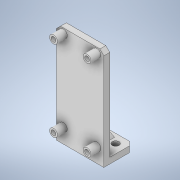
# Autodesk Inventor part: Vertical Ultrasonic Sensor Mount
Saved by Autodesk Inventor 2022.6 (Build 266554000, 554)
## iProperties
Created: 2024-10-19
Part Number: Vertical Ultrasonic Sensor Mount
Material: Generic
Document SubType Name: Modeling
Designer: Asus
Density: 1 g/cm^3
Appearance: Default
Author: Asus
Autodesk Inventor part; units mm, degrees
ref_plane "XY Plane" through (0, 0, 0) normal (0, 0, 1) x (1, 0, 0)
sketch "Sketch1" plane through (0, 0, 0) normal (0, 0, 1) x (1, 0, 0)
  line L0 (0, 0) -> (24, 0)
  line L1 (24, 0) -> (24, 46)
  line L2 (24, 46) -> (0, 46)
  line L3 (0, 46) -> (0, 0)
  line L4 (0, 46) -> (24, 46)
  line L5 (24, 46) -> (24, 46)
  line L6 (24, 46) -> (0, 46)
  line L7 (0, 46) -> (0, 46)
  dimension "d0" = 24
  dimension "d1" = 46
  dimension "d47" = 0
  dimension "d48" = 24
  constraints: 16 end point, 4 equal length, 2 horizontal, 2 perpendicular
  measures "d0" distance of L2.end L1.end
  measures "d1" distance of L1.end L0.end
  measures "d47" distance between parallel lines of L2 L6
  measures "d48" distance of L5.end L6.end
extrude "Extrusion1" add sketch "Sketch1" along normal blind 3
ref_plane "Work Plane1" through (12, 0, 0) normal (1, 0, 0) x (0, 1, 0)
ref_plane "Work Plane2" through (0, 23, 0) normal (0, 1, 0) x (-1, 0, 0)
sketch "Sketch2" plane through (0, 0, 3) normal (0, 0, 1) x (1, 0, 0)
  line L0 (24, 46) -> (0, 46) projected
  line L1 (0, 46) -> (0, 0) projected
  line L2 (24, 0) -> (24, 46) projected
  line L3 (0, 0) -> (24, 0) projected
  circle A0 centre (3.5, 43.5) radius 2
  circle A1 centre (3.5, 43.5) radius 1.2
  circle A2 centre (20.5, 43.5) radius 2
  circle A3 centre (20.5, 43.5) radius 1.2
  circle A4 centre (3.5, 2.5) radius 2
  circle A5 centre (3.5, 2.5) radius 1.2
  circle A6 centre (20.5, 2.5) radius 1.2
  circle A7 centre (20.5, 2.5) radius 2
  dimension "d4" = 17
  dimension "d6" = 41
  dimension "d7" = 2.5
  dimension "d8" = 3.5
  dimension "d11" = 3.5
  dimension "d12" = 3.5
  dimension "d13" = 2.5
  dimension "d14" = 41
  dimension "d15" = 4
  dimension "d16" = 2.4
  dimension "d17" = 4
  dimension "d18" = 2.4
  dimension "d19" = 4
  dimension "d20" = 2.4
  dimension "d21" = 2.4
  dimension "d22" = 4
  constraints: 8 centre point, 8 coincident
  measures "d4" distance of point (20.5, 43.5) point (3.5, 43.5)
  measures "d6" distance of point (3.5, 2.5) point (3.5, 43.5)
  measures "d7" distance from line of point (3.5, 43.5) L0
  measures "d8" distance from line of point (3.5, 43.5) L1
  measures "d11" distance from line of L1 point (3.5, 2.5)
  measures "d12" distance from line of L2 point (20.5, 2.5)
  measures "d13" distance from line of L3 point (20.5, 2.5)
  measures "d14" distance of point (20.5, 2.5) point (20.5, 43.5)
  measures "d15" diameter of A0
  measures "d16" diameter of A1
  measures "d17" diameter of A2
  measures "d18" diameter of A3
  measures "d19" diameter of A4
  measures "d20" diameter of A5
  measures "d21" diameter of A6
  measures "d22" diameter of A7
extrude "Extrusion2" add sketch "Sketch2" along normal blind 5 contours A0 | A2 | A4 | A7
hole "Hole1" at (3.5, 43.5, 3) at (20.5, 43.5, 3) at (3.5, 2.5, 3) at (20.5, 2.5, 3) direction (0, 0, -1) diameter 2.4 end through all
sketch "Sketch5" plane through (0, 46, 0) normal (0, 1, 0) x (1, 0, 0)
  line L0 (0, 0) -> (0, -3) projected
  line L1 (24, 0) -> (24, -3) projected
  line L2 (0, 0) -> (24, 0)
  line L3 (24, 0) -> (24, -3)
  line L4 (24, -3) -> (0, -3)
  line L5 (0, -3) -> (0, 0)
  constraints: 8 end point, 2 parallel, 1 horizontal, 1 perpendicular
extrude "Extrusion4" add sketch "Sketch5" along normal blind 5
sketch "Sketch6" plane through (0, 0, 3) normal (0, 0, 1) x (1, 0, 0)
  line L0 (0, 0) -> (0, 51) projected
  line L1 (24, 0) -> (24, 51) projected
  line L2 (0, 51) -> (24, 51)
  line L3 (24, 51) -> (24, 48)
  line L4 (24, 48) -> (0, 48)
  line L5 (0, 48) -> (0, 51)
  point P0 (0, 48)
  dimension "d51" = 3
  constraints: 8 end point, 2 parallel, 1 horizontal, 1 perpendicular, 1 point on line
  measures "d51" distance of L2.end L3.end
extrude "Extrusion5" add sketch "Sketch6" against normal blind 15
sketch "Sketch7" plane through (0, 51, 0) normal (0, 1, 0) x (1, 0, 0)
  line L0 (0, -3) -> (0, 12) projected
  line L1 (0, 12) -> (24, 12) projected
  line L2 (4.5, 7.5) -> (19.5, 7.5) construction
  line L3 (0, 0) -> (24, 0) projected
  point P0 (12, 7.5)
  dimension "d54" = 15
  dimension "d55" = 4.5
  dimension "d56" = 4.5
  constraints: 2 end point, 1 horizontal, 1 midpoint
  measures "d54" distance of L2.end L2.start
  measures "d55" distance from line of L2.start L0
  measures "d56" distance from line of L1 L2.start
hole "Hole3" at (4.5, 51, -7.5) at (19.5, 51, -7.5) direction (0, -1, 0) diameter 3.4 end through all
chamfer "Chamfer1" distance 2 angle 45 4 edges at (0, 49.5, -12) (24, 49.5, -12) (24, 0, 1.5) (0, 0, 1.5)
sketch "Sketch10" plane through (12, 0, 0) normal (1, 0, 0) x (0, 1, 0)
  line L0 (2, 3) -> (2, 0) projected
  line L1 (2, 3) -> (51, 3) projected
  line L2 (51, 3) -> (51, -10) projected
  line L3 (48, -10) -> (51, -10) projected
  line L4 (48, 0) -> (48, -10) projected
  line L5 (2, 0) -> (48, 0) projected
  line L6 (51, -10) -> (51, -12) projected
  line L7 (51, -12) -> (48, -12) projected
  line L8 (48, -12) -> (48, -10) projected
  line L9 (48, -10) -> (51, -10) projected
  line L10 (2, 0) -> (48, 0) projected
  line L11 (48, 0) -> (48, -10) projected
  line L12 (48, -10) -> (50.9713, -10)
  line L13 (48, -12) -> (48, -10) projected
  line L14 (48, -10) -> (18, 0)
  point P0 (0, 0)
  dimension "d74" = 30
  constraints: 4 end point, 1 point on line
  measures "d74" distance from line of L4 L14.end
extrude "Rib1" add sketch "Sketch10" along normal mid plane 5 rib yes fills toward (33.0158, -4.9526) open curves L14
chamfer "Chamfer3" distance 2 angle 45 4 edges at (14.5, 33, 0) (9.5, 33, 0) (9.5, 48, -5) (14.5, 48, -5)
body "Solid1"
